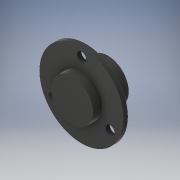
# Autodesk Inventor part: Slip Ring
Saved by Autodesk Inventor 2017 (Build 210142000, 142)
## iProperties
Created: 2018-10-22
Part Number: Slip Ring
Material: ABS Plastic
Document SubType Name: Modeling
Designer: Dell
Density: 1.06 g/cm^3
Appearance: Smooth - Black
Author: Dell
Autodesk Inventor part; units mm, degrees
ref_plane "YZ Plane" through (0, 0, 0) normal (1, 0, 0) x (0, 1, 0)
ref_plane "XZ Plane" through (0, 0, 0) normal (0, 1, 0) x (-1, 0, 0)
ref_plane "XY Plane" through (0, 0, 0) normal (0, 0, 1) x (1, 0, 0)
sketch "Sketch1" plane through (0, 0, 0) normal (0, 0, 1) x (1, 0, 0)
  circle A0 centre (0, 0) radius 11
  dimension "d0" = 22
  constraints: 1 centre point, 1 coincident
  measures "d0" diameter of A0
extrude "Extrusion1" add sketch "Sketch1" along normal blind 19
ref_plane "Work Plane1" through (0, 0, 14) normal (0, 0, 1) x (1, 0, 0)
sketch "Sketch2" plane through (0, 0, 14) normal (0, 0, 1) x (1, 0, 0)
  circle A0 centre (0, 0) radius 22.25
  circle A1 centre (0, 17.5) radius 2.5
  circle A2 centre (-15.1554, -8.75) radius 2.5
  circle A3 centre (15.1554, -8.75) radius 2.5
  dimension "d4" = 44.5
  dimension "d5" = 5
  dimension "d6" = 17.5
  dimension "d9" = 360
  constraints: 4 centre point, 1 coincident, 1 vertical alignment, 7 other
  measures "d4" diameter of A0
  measures "d5" diameter of A1
  measures "d6" distance of point (0, 0) A1.centre
extrude "Extrusion2" add sketch "Sketch2" against normal blind 2.3
body "Solid1"
